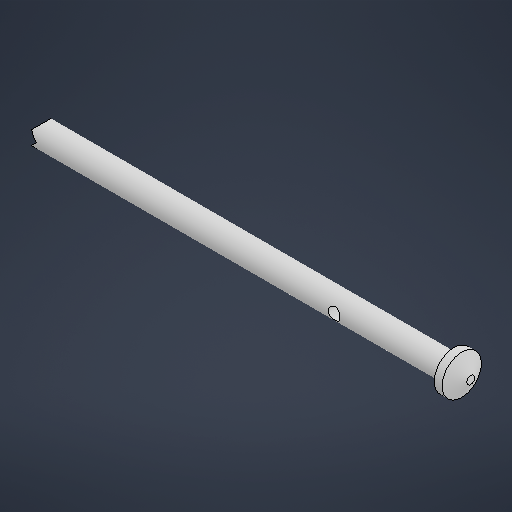
# Autodesk Inventor part: TW1-002
Saved by Autodesk Inventor 2025.3 (Build 293356000, 356)
## iProperties
Created: 2025-05-04
Part Number: TW1-002
Material: Generic
Document SubType Name: Modeling
Designer: fablabadmin
Density: 1 g/cm^3
Appearance: Default
Description: Plunger
Stock Number: C45E
Author: Benjamin Solar
Title: WEDU
Revision Number: 1
Autodesk Inventor part; units mm, degrees
ref_plane "YZ Plane" through (0, 0, 0) normal (1, 0, 0) x (0, 1, 0)
ref_plane "XZ Plane" through (0, 0, 0) normal (0, 1, 0) x (-1, 0, 0)
ref_plane "XY Plane" through (0, 0, 0) normal (0, 0, 1) x (1, 0, 0)
sketch "Sketch1" plane through (0, 0, 0) normal (0, 0, 1) x (1, 0, 0)
  line L0 (-22.3155, 0) -> (133.8928, 0) projected
  line L1 (0, -4.6) -> (0, 6.6) projected
  line L2 (0, 3) -> (106.6906, 3)
  line L3 (106.6906, 3) -> (106.6906, 5)
  line L4 (106.6906, 5) -> (108.6906, 5)
  line L5 (108.6906, 5) -> (111.5774, 0)
  line L6 (0, 3) -> (3, 0)
  line L7 (0, 3) -> (0, 0)
  line L8 (111, 1) -> (111, 0)
  line L9 (0, -3) -> (3, 0)
  circle A0 centre (79.02, 0) radius 1.5
  line L10 (2.5, 3) -> (1.25, 1.75)
  line L11 (0, -3) -> (106.6906, -3)
  line L12 (2.5, -3) -> (1.25, -1.75)
  dimension "d0" = 6
  dimension "d1" = 3
  dimension "d2" = 60
  dimension "d3" = 2
  dimension "d4" = 10
  dimension "d5" = 2
  dimension "d6" = 111
  dimension "d10" = 3
  dimension "d14" = 2.5
  dimension "d16" = 31.98
  constraints: 22 end point, 9 point on line, 5 perpendicular, 4 symmetric about line, 1 centre point, 1 collinear
  measures "d0" diameter of L2 L0
  measures "d1" horizontal distance of L6.end L2.start
  measures "d2" angle of L0 L5
  measures "d3" diameter of L8.start L0
  measures "d4" diameter of L4 L0
  measures "d5" distance of L3.end L4.end
  measures "d6" distance between parallel lines of L8 L1
  measures "d10" diameter of A0
  measures "d14" distance of L2.start L10.start
  measures "d16" horizontal distance of A0.centre L8.start
revolve "Revolution1" add sketch "Sketch1" angle 360 about axis through (-10, 0, 0) along (1, 0, 0) picked at (79.1973, 0.4675) contours L6 L10 L2 L3 L4 L5 L8 L0 A0 | L2 L10 L6 | A0 L0
extrude "Extrusion1" cut sketch "Sketch1" along normal through all both and the other way through all contours L1 L6 L0 | L0 L9 L1 | L9 L12 L11 | L2 L10 L6 | A0 L0 | L0 A0
equation "\"d1\" = 0.5 * d0"
body "Solid1"
